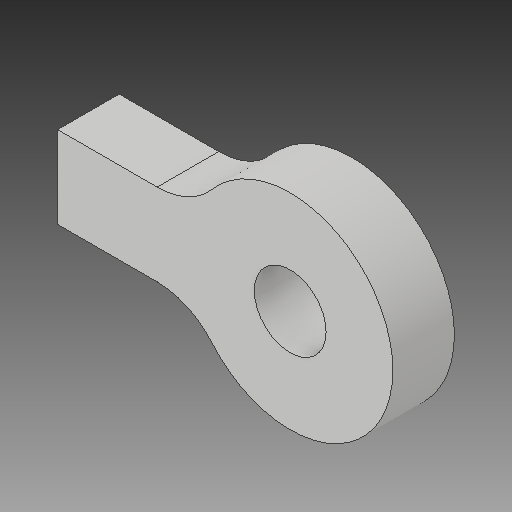
# Autodesk Inventor part: Anillo riel
Saved by Autodesk Inventor 2019 (Build 230136000, 136)
## iProperties
Created: 2020-02-01
Part Number: Anillo riel
Material: Generic
Document SubType Name: Modeling
Designer: Elías Sánchez
Density: 1 g/cm^3
Appearance: Default
Description: Corte Láser
Author: Elías Sánchez
Autodesk Inventor part; units mm, degrees
ref_plane "YZ Plane" through (0, 0, 0) normal (1, 0, 0) x (0, 1, 0)
ref_plane "XZ Plane" through (0, 0, 0) normal (0, 1, 0) x (-1, 0, 0)
ref_plane "XY Plane" through (0, 0, 0) normal (0, 0, 1) x (1, 0, 0)
sketch "Sketch1" plane through (0, 0, 0) normal (0, 0, 1) x (1, 0, 0)
  line L0 (0, 0) -> (13.5, 0)
  line L1 (13.5, 8) -> (0, 8)
  line L2 (0, 8) -> (0, 0)
  arc A0 (13.5, 0) -> (13.5, 8) centre (22.6652, 4) ccw
  circle A1 centre (22.6652, 4) radius 3.5
  dimension "d0" = 8
  dimension "d2" = 10
  dimension "d5" = 7
  dimension "d10" = 4
  dimension "d12" = 13.5
  constraints: 6 end point, 2 centre point, 2 point on circle, 1 coincident, 1 horizontal, 1 parallel, 1 vertical
  measures "d0" distance of L1.end L0.start
  measures "d2" radius of A0
  measures "d5" diameter of A1
  measures "d10" distance from line of L0 A0.centre
  measures "d12" distance of L0.start L0.end
extrude "Extrusion1" add sketch "Sketch1" along normal blind 6
fillet "Fillet1" radius 7 2 edges at (13.5, 8, 3) (13.5, 0, 3)
equation "\"d10\" = 0.5 * d0"
body "Solid1"
